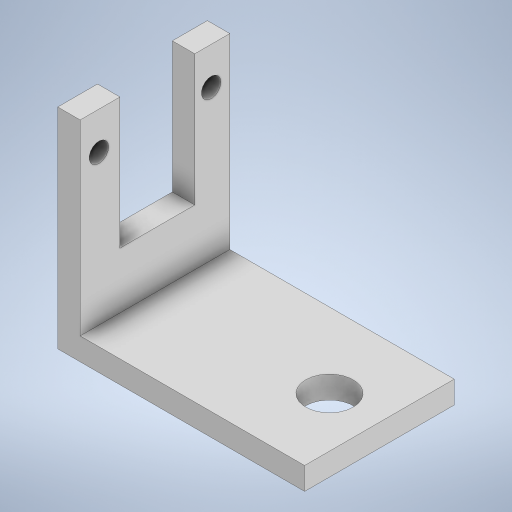
# Autodesk Inventor part: motor_angle
Saved by Autodesk Inventor 2023 (Build 270158000, 158)
## iProperties
Created: 2023-04-09
Part Number: motor_angle
Material: Generic
Document SubType Name: Modeling
Designer: Nikhil
Density: 1 g/cm^3
Appearance: Default
Author: Nikhil
Autodesk Inventor part; units mm, degrees
ref_plane "YZ Plane" through (0, 0, 0) normal (1, 0, 0) x (0, 1, 0)
ref_plane "XZ Plane" through (0, 0, 0) normal (0, 1, 0) x (-1, 0, 0)
ref_plane "XY Plane" through (0, 0, 0) normal (0, 0, 1) x (1, 0, 0)
sketch "Sketch1" plane through (0, 0, 0) normal (0, 0, 1) x (1, 0, 0)
  line L0 (0, 0) -> (0, 56)
  line L1 (0, 56) -> (6, 56)
  line L2 (6, 56) -> (6, 6)
  line L3 (6, 6) -> (66, 6)
  line L4 (66, 6) -> (66, 0)
  line L5 (66, 0) -> (0, 0)
  dimension "d0" = 56
  dimension "d1" = 6
  dimension "d2" = 50
  dimension "d3" = 60
  dimension "d4" = 6
  constraints: 12 end point, 3 perpendicular, 1 horizontal, 1 vertical
  measures "d0" distance of L0.start L0.end
  measures "d1" distance of L0.end L1.end
  measures "d2" distance of L1.end L2.end
  measures "d3" distance of L2.end L3.end
  measures "d4" distance of L3.end L4.end
extrude "Extrusion1" add sketch "Sketch1" along normal blind 40
sketch "Sketch2" plane through (6, 6, 0) normal (0, 1, 0) x (1, 0, 0)
  line L0 (0, 0) -> (0, -40) projected
  circle A0 centre (46.65, -20) radius 6.35
  line L1 (60, 0) -> (0, 0) projected
  line L2 (60, -40) -> (0, -40) projected
  point P0 (-6, 0)
  dimension "d8" = 12.7
  dimension "d25" = 46.65
  constraints: 1 centre point, 1 coincident
  measures "d8" diameter of A0
  measures "d25" distance from line of A0.centre L0
extrude "Extrusion2" cut sketch "Sketch2" against normal blind 40
sketch "Sketch3" plane through (6, 6, 0) normal (1, 0, 0) x (0, 0, -1)
  line L0 (0, 50) -> (-40, 50) projected
  line L1 (-29.3643, 50) -> (-9.3643, 50)
  line L2 (-9.3643, 50) -> (-9.3643, 15)
  line L3 (-9.3643, 15) -> (-29.3643, 15)
  line L4 (-29.3643, 15) -> (-29.3643, 50)
  point P0 (0, -6)
  dimension "d13" = 20
  dimension "d14" = 35
  constraints: 8 end point, 2 parallel, 1 horizontal, 1 perpendicular, 1 point on line
  measures "d13" distance of L2.end L3.end
  measures "d14" distance of L1.end L2.end
extrude "Extrusion3" cut sketch "Sketch3" against normal blind 10
sketch "Sketch4" plane through (6, 6, 0) normal (1, 0, 0) x (0, 0, -1)
  circle A0 centre (-35, 40) radius 2.6
  line L0 (-40, 0) -> (-40, 50) projected
  line L1 (-29.3643, 50) -> (-40, 50) projected
  point P0 (0, -6)
  dimension "d17" = 5.2
  dimension "d18" = 5
  dimension "d19" = 10
  constraints: 1 centre point
  measures "d17" diameter of A0
  measures "d18" distance from line of L0 A0.centre
  measures "d19" distance from line of A0.centre L1
extrude "Extrusion4" cut sketch "Sketch4" against normal blind 10
pattern_linear "Rectangular Pattern1" count 2 spacing 30 along (0, 0, -1) of "Extrusion4"
body "Solid1"
